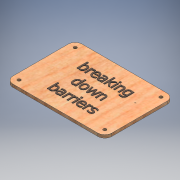
# Autodesk Inventor part: PromptPanel
Saved by Autodesk Inventor 2016 (Build 200138000, 138)
## iProperties
Created: 2015-09-18
Part Number: PromptPanel
Material: Generic
Document SubType Name: Modeling
Designer: Erin
Density: 1 g/cm^3
Appearance: Default
Author: Erin
Autodesk Inventor part; units mm, degrees
(part 1 of 2)
ref_plane "YZ Plane" through (0, 0, 0) normal (1, 0, 0) x (0, 1, 0)
ref_plane "XZ Plane" through (0, 0, 0) normal (0, 1, 0) x (-1, 0, 0)
ref_plane "XY Plane" through (0, 0, 0) normal (0, 0, 1) x (1, 0, 0)
derived "FrontPanel.ipt"
sketch "Sketch1" plane through (0, 0, 0) normal (0, 0, 1) x (1, 0, 0)
  line L0 (-60, 85) -> (60, 85)
  line L1 (60, 85) -> (60, -85)
  line L2 (60, -85) -> (-60, -85)
  line L3 (-60, -85) -> (-60, 85)
  line L4 (-50, 56.6301) -> (50, 56.6301)
  line L5 (50, 56.6301) -> (50, -13.3699)
  line L6 (50, -13.3699) -> (-50, -13.3699)
  line L7 (-50, -13.3699) -> (-50, 56.6301)
  circle A0 centre (-25, -55) radius 13.85
  circle A1 centre (-25, -24.425) radius 2.7
  circle A2 centre (25, -24.425) radius 2.7
  line L8 (-25, 85) -> (-25, -85) construction
  line L9 (-60, -55) -> (60, -55) construction
  circle A3 centre (-25, -55) radius 17.875 construction
  line L10 (25, 85) -> (25, -85) construction
  circle A4 centre (25, -55) radius 13.85
  circle A5 centre (25, -55) radius 17.875 construction
  circle A6 centre (-53.4, -78.4) radius 1.6
  line L11 (-52.9471, 75) -> (52.9471, 75) construction
  line L12 (52.9471, 75) -> (52.9471, 66.6301) construction
  line L13 (52.9471, 66.6301) -> (-52.9471, 66.6301) construction
  line L14 (-52.9471, 66.6301) -> (-52.9471, 75) construction
  circle A7 centre (-43.4, -6.7699) radius 1.6
  line L15 (-50, 21.6301) -> (50, 21.6301) construction
  line L16 (0, 56.6301) -> (0, -13.3699) construction
  circle A8 centre (-43.4, 50.0301) radius 1.6
  circle A9 centre (43.4, 50.0301) radius 1.6
  circle A10 centre (43.4, -6.7699) radius 1.6
  line L17 (-60, 0) -> (60, 0) construction
  circle A11 centre (53.4, -78.4) radius 1.6
  circle A12 centre (53.4, 78.4) radius 1.6
  circle A13 centre (-53.4, 78.4) radius 1.6
  point P0 (0, 0)
  point P1 (0, 85)
  point P2 (0, 75)
extrude "Extrusion1" add sketch "Sketch1" along normal blind 3 contours L4 L5 L6 L7
fillet "Fillet1" radius 7 4 edges at (-50, -13.3699, 1.5) (-50, 56.6301, 1.5) (50, 56.6301, 1.5) (50, -13.3699, 1.5)
sketch "Sketch2" plane through (-43, 56.6301, 3) normal (0, 0, 1) x (1, 0, 0)
  line L0 (25.4474, -13.3812) -> (62.0414, -13.3812) construction
  line L1 (62.0414, -13.3812) -> (62.0414, -43.8913) construction
  line L2 (62.0414, -43.8913) -> (25.4474, -43.8913) construction
  line L3 (25.4474, -43.8913) -> (25.4474, -13.3812) construction
  spline S0 degree 2 poles (24.8101, -19.9533) (24.8101, -21.7928) (23.0272, -24.0376) (21.682, -24.0376) knots 0 0 0 1 2 2 2
  spline S1 degree 2 poles (21.682, -24.0376) (21.0742, -24.0376) (20.2071, -23.7377) (19.7857, -23.4784) knots 0 0 0 1 2 2 2
  line L4 (19.7857, -23.4784) -> (19.7047, -23.8269)
  line L5 (19.7047, -23.8269) -> (18.5216, -23.8269)
  line L6 (18.5216, -23.8269) -> (18.5216, -13.3812)
  line L7 (18.5216, -13.3812) -> (19.7857, -13.3812)
  line L8 (19.7857, -13.3812) -> (19.7857, -17.1089)
  spline S2 degree 2 poles (19.7857, -17.1089) (20.2639, -16.6794) (21.3741, -16.1121) (22.0791, -16.1121) knots 0 0 0 1 2 2 2
  spline S3 degree 2 poles (22.0791, -16.1121) (23.3514, -16.1121) (24.8101, -18.1462) (24.8101, -19.9533) knots 0 0 0 1 2 2 2
  spline S4 degree 2 poles (23.5054, -20.0505) (23.5054, -18.7053) (22.6869, -17.3115) (21.7793, -17.3115) knots 0 0 0 1 2 2 2
  spline S5 degree 2 poles (21.7793, -17.3115) (21.2687, -17.3115) (20.2152, -17.7977) (19.7857, -18.1705) knots 0 0 0 1 2 2 2
  line L9 (19.7857, -18.1705) -> (19.7857, -22.4735)
  spline S6 degree 2 poles (19.7857, -22.4735) (20.2639, -22.7085) (21.0013, -22.903) (21.4389, -22.903) knots 0 0 0 1 2 2 2
  spline S7 degree 2 poles (21.4389, -22.903) (22.4032, -22.903) (23.5054, -21.5335) (23.5054, -20.0505) knots 0 0 0 1 2 2 2
  line L10 (30.1018, -17.6761) -> (30.037, -17.6761)
  spline S8 degree 2 poles (30.037, -17.6761) (29.8911, -17.6356) (29.575, -17.6194) (29.3562, -17.6194) knots 0 0 0 1 2 2 2
  spline S9 degree 2 poles (29.3562, -17.6194) (28.8457, -17.6194) (27.8408, -18.0651) (27.387, -18.5027) knots 0 0 0 1 2 2 2
  line L11 (27.387, -18.5027) -> (27.387, -23.8269)
  line L12 (27.387, -23.8269) -> (26.1229, -23.8269)
  line L13 (26.1229, -23.8269) -> (26.1229, -16.3228)
  line L14 (26.1229, -16.3228) -> (27.387, -16.3228)
  line L15 (27.387, -16.3228) -> (27.387, -17.4411)
  spline S10 degree 2 poles (27.387, -17.4411) (28.0759, -16.8252) (29.105, -16.3228) (29.5913, -16.3228) knots 0 0 0 1 2 2 2
  spline S11 degree 2 poles (29.5913, -16.3228) (29.7857, -16.3228) (29.9802, -16.339) (30.1018, -16.3633) knots 0 0 0 1 2 2 2
  line L16 (30.1018, -16.3633) -> (30.1018, -17.6761)
  spline S12 degree 2 poles (34.34, -23.997) (32.541, -23.997) (30.5637, -21.9792) (30.5637, -20.1154) knots 0 0 0 1 2 2 2
  spline S13 degree 2 poles (30.5637, -20.1154) (30.5637, -18.2839) (32.4843, -16.1121) (34.0321, -16.1121) knots 0 0 0 1 2 2 2
  spline S14 degree 2 poles (34.0321, -16.1121) (34.729, -16.1121) (35.8068, -16.5173) (36.2039, -16.9468) knots 0 0 0 1 2 2 2
  spline S15 degree 2 poles (36.2039, -16.9468) (36.6091, -17.3763) (37.0386, -18.6162) (37.0386, -19.5157) knots 0 0 0 1 2 2 2
  line L17 (37.0386, -19.5157) -> (37.0386, -20.2045)
  line L18 (37.0386, -20.2045) -> (31.8441, -20.2045)
  spline S16 degree 2 poles (31.8441, -20.2045) (31.8441, -21.5092) (33.1569, -22.8949) (34.3238, -22.8949) knots 0 0 0 1 2 2 2
  spline S17 degree 2 poles (34.3238, -22.8949) (34.7371, -22.8949) (35.5394, -22.7085) (35.8635, -22.5627) knots 0 0 0 1 2 2 2
  spline S18 degree 2 poles (35.8635, -22.5627) (36.2039, -22.4006) (36.6739, -22.117) (36.8279, -21.9873) knots 0 0 0 1 2 2 2
  line L19 (36.8279, -21.9873) -> (36.9008, -21.9873)
  line L20 (36.9008, -21.9873) -> (36.9008, -23.365)
  spline S19 degree 2 poles (36.9008, -23.365) (36.682, -23.4541) (36.0175, -23.7134) (35.7582, -23.7863) knots 0 0 0 1 2 2 2
  spline S20 degree 2 poles (35.7582, -23.7863) (35.3935, -23.8917) (34.7938, -23.997) (34.34, -23.997) knots 0 0 0 1 2 2 2
  spline S21 degree 2 poles (35.8068, -19.2402) (35.7906, -18.7296) (35.5799, -17.9841) (35.3773, -17.7329) knots 0 0 0 1 2 2 2
  spline S22 degree 2 poles (35.3773, -17.7329) (35.1585, -17.4492) (34.4697, -17.1494) (33.9592, -17.1494) knots 0 0 0 1 2 2 2
  spline S23 degree 2 poles (33.9592, -17.1494) (33.4567, -17.1494) (32.7517, -17.4492) (32.46, -17.741) knots 0 0 0 1 2 2 2
  spline S24 degree 2 poles (32.46, -17.741) (32.1763, -18.0408) (31.8846, -18.762) (31.8441, -19.2402) knots 0 0 0 1 2 2 2
  line L21 (31.8441, -19.2402) -> (35.8068, -19.2402)
  spline S25 degree 2 poles (42.5005, -23.0327) (42.3465, -23.1462) (41.8279, -23.5513) (41.5848, -23.6729) knots 0 0 0 1 2 2 2
  spline S26 degree 2 poles (41.5848, -23.6729) (41.2525, -23.8512) (40.6285, -24.0376) (40.0613, -24.0376) knots 0 0 0 1 2 2 2
  spline S27 degree 2 poles (40.0613, -24.0376) (39.5994, -24.0376) (38.7647, -23.6891) (38.4486, -23.3731) knots 0 0 0 1 2 2 2
  spline S28 degree 2 poles (38.4486, -23.3731) (38.1488, -23.0651) (37.7841, -22.1575) (37.7841, -21.6551) knots 0 0 0 1 2 2 2
  spline S29 degree 2 poles (37.7841, -21.6551) (37.7841, -20.8771) (38.4405, -19.775) (39.1537, -19.459) knots 0 0 0 1 2 2 2
  spline S30 degree 2 poles (39.1537, -19.459) (39.7857, -19.1672) (41.5037, -18.9484) (42.5005, -18.8917) knots 0 0 0 1 2 2 2
  line L22 (42.5005, -18.8917) -> (42.5005, -18.6486)
  spline S31 degree 2 poles (42.5005, -18.6486) (42.5005, -18.211) (42.2331, -17.668) (41.99, -17.5141) knots 0 0 0 1 2 2 2
  spline S32 degree 2 poles (41.99, -17.5141) (41.7468, -17.3601) (41.0499, -17.2628) (40.6772, -17.2628) knots 0 0 0 1 2 2 2
  spline S33 degree 2 poles (40.6772, -17.2628) (40.2396, -17.2628) (39.0564, -17.5222) (38.4648, -17.7734) knots 0 0 0 1 2 2 2
  line L23 (38.4648, -17.7734) -> (38.3919, -17.7734)
  line L24 (38.3919, -17.7734) -> (38.3919, -16.4849)
  spline S34 degree 2 poles (38.3919, -16.4849) (38.7404, -16.3876) (40.0451, -16.1445) (40.6853, -16.1445) knots 0 0 0 1 2 2 2
  spline S35 degree 2 poles (40.6853, -16.1445) (41.4632, -16.1445) (42.5248, -16.3876) (42.9462, -16.7037) knots 0 0 0 1 2 2 2
  spline S36 degree 2 poles (42.9462, -16.7037) (43.3595, -17.0116) (43.7647, -17.9922) (43.7647, -18.6972) knots 0 0 0 1 2 2 2
  line L25 (43.7647, -18.6972) -> (43.7647, -23.8269)
  line L26 (43.7647, -23.8269) -> (42.5005, -23.8269)
  line L27 (42.5005, -23.8269) -> (42.5005, -23.0327)
  line L28 (42.5005, -21.9792) -> (42.5005, -19.8966)
  spline S37 degree 2 poles (42.5005, -19.8966) (42.0467, -19.9371) (40.6772, -20.0748) (40.2477, -20.2045) knots 0 0 0 1 2 2 2
  spline S38 degree 2 poles (40.2477, -20.2045) (39.7452, -20.3585) (39.0888, -20.9987) (39.0888, -21.5659) knots 0 0 0 1 2 2 2
  spline S39 degree 2 poles (39.0888, -21.5659) (39.0888, -22.2142) (39.8182, -22.8706) (40.5151, -22.8706) knots 0 0 0 1 2 2 2
  spline S40 degree 2 poles (40.5151, -22.8706) (41.1066, -22.8706) (42.0791, -22.3601) (42.5005, -21.9792) knots 0 0 0 1 2 2 2
  line L29 (51.7549, -23.8269) -> (50.0937, -23.8269)
  line L30 (50.0937, -23.8269) -> (47.306, -20.2045)
  line L31 (47.306, -20.2045) -> (46.8036, -20.6907)
  line L32 (46.8036, -20.6907) -> (46.8036, -23.8269)
  line L33 (46.8036, -23.8269) -> (45.5394, -23.8269)
  line L34 (45.5394, -23.8269) -> (45.5394, -13.3812)
  line L35 (45.5394, -13.3812) -> (46.8036, -13.3812)
  line L36 (46.8036, -13.3812) -> (46.8036, -19.4914)
  line L37 (46.8036, -19.4914) -> (49.7695, -16.3228)
  line L38 (49.7695, -16.3228) -> (51.3417, -16.3228)
  line L39 (51.3417, -16.3228) -> (48.2622, -19.459)
  line L40 (48.2622, -19.459) -> (51.7549, -23.8269)
  line L41 (53.6755, -23.8269) -> (52.4113, -23.8269)
  line L42 (52.4113, -23.8269) -> (52.4113, -16.3228)
  line L43 (52.4113, -16.3228) -> (53.6755, -16.3228)
  line L44 (53.6755, -16.3228) -> (53.6755, -23.8269)
  line L45 (53.7647, -15.0748) -> (52.3303, -15.0748)
  line L46 (52.3303, -15.0748) -> (52.3303, -13.762)
  line L47 (52.3303, -13.762) -> (53.7647, -13.762)
  line L48 (53.7647, -13.762) -> (53.7647, -15.0748)
  line L49 (61.4227, -23.8269) -> (60.1585, -23.8269)
  line L50 (60.1585, -23.8269) -> (60.1585, -19.5481)
  spline S41 degree 2 poles (60.1585, -19.5481) (60.1585, -19.0295) (60.0613, -18.138) (59.9154, -17.8706) knots 0 0 0 1 2 2 2
  spline S42 degree 2 poles (59.9154, -17.8706) (59.7614, -17.587) (59.2104, -17.3115) (58.7404, -17.3115) knots 0 0 0 1 2 2 2
  spline S43 degree 2 poles (58.7404, -17.3115) (58.2703, -17.3115) (57.2736, -17.8139) (56.7955, -18.2191) knots 0 0 0 1 2 2 2
  line L51 (56.7955, -18.2191) -> (56.7955, -23.8269)
  line L52 (56.7955, -23.8269) -> (55.5313, -23.8269)
  line L53 (55.5313, -23.8269) -> (55.5313, -16.3228)
  line L54 (55.5313, -16.3228) -> (56.7955, -16.3228)
  line L55 (56.7955, -16.3228) -> (56.7955, -17.1575)
  spline S44 degree 2 poles (56.7955, -17.1575) (57.3627, -16.647) (58.4567, -16.1121) (59.0726, -16.1121) knots 0 0 0 1 2 2 2
  spline S45 degree 2 poles (59.0726, -16.1121) (60.1747, -16.1121) (61.4227, -17.5708) (61.4227, -18.9565) knots 0 0 0 1 2 2 2
  line L56 (61.4227, -18.9565) -> (61.4227, -23.8269)
  spline S46 degree 2 poles (63.4648, -25.0262) (63.5945, -25.0829) (64.0888, -25.2612) (64.4049, -25.3342) knots 0 0 0 1 2 2 2
  spline S47 degree 2 poles (64.4049, -25.3342) (64.7533, -25.4233) (65.3449, -25.5286) (65.6934, -25.5286) knots 0 0 0 1 2 2 2
  spline S48 degree 2 poles (65.6934, -25.5286) (66.2768, -25.5286) (67.0872, -25.2207) (67.3141, -24.9452) knots 0 0 0 1 2 2 2
  spline S49 degree 2 poles (67.3141, -24.9452) (67.5329, -24.6697) (67.7031, -23.9484) (67.7031, -23.4865) knots 0 0 0 1 2 2 2
  line L57 (67.7031, -23.4865) -> (67.7031, -22.8301)
  spline S50 degree 2 poles (67.7031, -22.8301) (67.1925, -23.2758) (66.212, -23.6972) (65.4746, -23.6972) knots 0 0 0 1 2 2 2
  spline S51 degree 2 poles (65.4746, -23.6972) (64.1942, -23.6972) (62.6788, -21.7928) (62.6788, -20.0019) knots 0 0 0 1 2 2 2
  spline S52 degree 2 poles (62.6788, -20.0019) (62.6788, -19.07) (63.2055, -17.6275) (63.6431, -17.117) knots 0 0 0 1 2 2 2
  spline S53 degree 2 poles (63.6431, -17.117) (64.0645, -16.6389) (65.2233, -16.1121) (65.8392, -16.1121) knots 0 0 0 1 2 2 2
  spline S54 degree 2 poles (65.8392, -16.1121) (66.4227, -16.1121) (67.2736, -16.3876) (67.7031, -16.6389) knots 0 0 0 1 2 2 2
  line L58 (67.7031, -16.6389) -> (67.776, -16.3228)
  line L59 (67.776, -16.3228) -> (68.9673, -16.3228)
  line L60 (68.9673, -16.3228) -> (68.9673, -22.9679)
  spline S55 degree 2 poles (68.9673, -22.9679) (68.9673, -24.8803) (67.306, -26.6632) (65.5961, -26.6632) knots 0 0 0 1 2 2 2
  spline S56 degree 2 poles (65.5961, -26.6632) (65.0451, -26.6632) (63.8943, -26.4849) (63.4, -26.339) knots 0 0 0 1 2 2 2
  line L61 (63.4, -26.339) -> (63.4, -25.0262)
  line L62 (63.4, -25.0262) -> (63.4648, -25.0262)
  line L63 (67.7031, -21.7928) -> (67.7031, -17.668)
  spline S57 degree 2 poles (67.7031, -17.668) (67.2331, -17.4411) (66.4389, -17.2466) (66.0418, -17.2466) knots 0 0 0 1 2 2 2
  spline S58 degree 2 poles (66.0418, -17.2466) (65.0856, -17.2466) (63.9835, -18.6567) (63.9835, -19.9776) knots 0 0 0 1 2 2 2
  spline S59 degree 2 poles (63.9835, -19.9776) (63.9835, -21.2256) (64.8182, -22.5303) (65.7582, -22.5303) knots 0 0 0 1 2 2 2
  spline S60 degree 2 poles (65.7582, -22.5303) (66.2525, -22.5303) (67.2898, -22.1413) (67.7031, -21.7928) knots 0 0 0 1 2 2 2
  line L64 (33.9632, -40.2916) -> (32.699, -40.2916)
  line L65 (32.699, -40.2916) -> (32.699, -39.5298)
  spline S61 degree 2 poles (32.699, -39.5298) (32.4073, -39.773) (31.9778, -40.0971) (31.6861, -40.2349) knots 0 0 0 1 2 2 2
  spline S62 degree 2 poles (31.6861, -40.2349) (31.4186, -40.3645) (30.8433, -40.5023) (30.4624, -40.5023) knots 0 0 0 1 2 2 2
  spline S63 degree 2 poles (30.4624, -40.5023) (29.8465, -40.5023) (28.8092, -39.9918) (28.4446, -39.4974) knots 0 0 0 1 2 2 2
  spline S64 degree 2 poles (28.4446, -39.4974) (28.0799, -39.0031) (27.6747, -37.5444) (27.6747, -36.5963) knots 0 0 0 1 2 2 2
  spline S65 degree 2 poles (27.6747, -36.5963) (27.6747, -35.6076) (28.1853, -34.1652) (28.631, -33.6222) knots 0 0 0 1 2 2 2
  spline S66 degree 2 poles (28.631, -33.6222) (29.0442, -33.136) (30.2031, -32.5769) (30.8433, -32.5769) knots 0 0 0 1 2 2 2
  spline S67 degree 2 poles (30.8433, -32.5769) (31.4024, -32.5769) (32.2371, -32.8281) (32.699, -33.0874) knots 0 0 0 1 2 2 2
  line L66 (32.699, -33.0874) -> (32.699, -29.8459)
  line L67 (32.699, -29.8459) -> (33.9632, -29.8459)
  line L68 (33.9632, -29.8459) -> (33.9632, -40.2916)
  line L69 (32.699, -38.4683) -> (32.699, -34.1328)
  spline S68 degree 2 poles (32.699, -34.1328) (32.229, -33.9059) (31.4835, -33.7357) (31.054, -33.7357) knots 0 0 0 1 2 2 2
  spline S69 degree 2 poles (31.054, -33.7357) (30.0815, -33.7357) (28.9794, -35.1944) (28.9794, -36.572) knots 0 0 0 1 2 2 2
  spline S70 degree 2 poles (28.9794, -36.572) (28.9794, -37.901) (29.8222, -39.3029) (30.7541, -39.3029) knots 0 0 0 1 2 2 2
  spline S71 degree 2 poles (30.7541, -39.3029) (31.2485, -39.3029) (32.2533, -38.8491) (32.699, -38.4683) knots 0 0 0 1 2 2 2
  spline S72 degree 2 poles (41.9616, -36.5396) (41.9616, -38.4358) (40.1383, -40.5023) (38.6148, -40.5023) knots 0 0 0 1 2 2 2
  spline S73 degree 2 poles (38.6148, -40.5023) (37.0507, -40.5023) (35.2598, -38.371) (35.2598, -36.5396) knots 0 0 0 1 2 2 2
  spline S74 degree 2 poles (35.2598, -36.5396) (35.2598, -34.6595) (37.1075, -32.5769) (38.6148, -32.5769) knots 0 0 0 1 2 2 2
  spline S75 degree 2 poles (38.6148, -32.5769) (40.1383, -32.5769) (41.9616, -34.6514) (41.9616, -36.5396) knots 0 0 0 1 2 2 2
  spline S76 degree 2 poles (40.6569, -36.5396) (40.6569, -35.0809) (39.5953, -33.6628) (38.6148, -33.6628) knots 0 0 0 1 2 2 2
  spline S77 degree 2 poles (38.6148, -33.6628) (37.6342, -33.6628) (36.5645, -35.0809) (36.5645, -36.5396) knots 0 0 0 1 2 2 2
  spline S78 degree 2 poles (36.5645, -36.5396) (36.5645, -37.9577) (37.6342, -39.4164) (38.6148, -39.4164) knots 0 0 0 1 2 2 2
  spline S79 degree 2 poles (38.6148, -39.4164) (39.5872, -39.4164) (40.6569, -37.982) (40.6569, -36.5396) knots 0 0 0 1 2 2 2
  line L70 (52.3506, -32.7875) -> (50.4462, -40.2916)
  line L71 (50.4462, -40.2916) -> (49.2793, -40.2916)
  line L72 (49.2793, -40.2916) -> (47.4478, -34.5055)
  line L73 (47.4478, -34.5055) -> (45.6245, -40.2916)
  line L74 (45.6245, -40.2916) -> (44.4656, -40.2916)
  line L75 (44.4656, -40.2916) -> (42.5451, -32.7875)
  line L76 (42.5451, -32.7875) -> (43.8579, -32.7875)
  line L77 (43.8579, -32.7875) -> (45.1869, -38.5979)
  line L78 (45.1869, -38.5979) -> (46.9616, -32.7875)
  line L79 (46.9616, -32.7875) -> (48.007, -32.7875)
  line L80 (48.007, -32.7875) -> (49.8303, -38.5979)
  line L81 (49.8303, -38.5979) -> (51.0783, -32.7875)
  line L82 (51.0783, -32.7875) -> (52.3506, -32.7875)
  line L83 (59.3522, -40.2916) -> (58.088, -40.2916)
  line L84 (58.088, -40.2916) -> (58.088, -36.0128)
  spline S80 degree 2 poles (58.088, -36.0128) (58.088, -35.4942) (57.9908, -34.6028) (57.8449, -34.3354) knots 0 0 0 1 2 2 2
  spline S81 degree 2 poles (57.8449, -34.3354) (57.6909, -34.0517) (57.1399, -33.7762) (56.6699, -33.7762) knots 0 0 0 1 2 2 2
  spline S82 degree 2 poles (56.6699, -33.7762) (56.1998, -33.7762) (55.2031, -34.2786) (54.725, -34.6838) knots 0 0 0 1 2 2 2
  line L85 (54.725, -34.6838) -> (54.725, -40.2916)
  line L86 (54.725, -40.2916) -> (53.4608, -40.2916)
  line L87 (53.4608, -40.2916) -> (53.4608, -32.7875)
  line L88 (53.4608, -32.7875) -> (54.725, -32.7875)
  line L89 (54.725, -32.7875) -> (54.725, -33.6222)
  spline S83 degree 2 poles (54.725, -33.6222) (55.2922, -33.1117) (56.3862, -32.5769) (57.0021, -32.5769) knots 0 0 0 1 2 2 2
  spline S84 degree 2 poles (57.0021, -32.5769) (58.1042, -32.5769) (59.3522, -34.0355) (59.3522, -35.4213) knots 0 0 0 1 2 2 2
  line L90 (59.3522, -35.4213) -> (59.3522, -40.2916)
  spline S85 degree 2 poles (27.8408, -52.8828) (27.8408, -54.7223) (26.058, -56.967) (24.7128, -56.967) knots 0 0 0 1 2 2 2
  spline S86 degree 2 poles (24.7128, -56.967) (24.105, -56.967) (23.2379, -56.6672) (22.8165, -56.4079) knots 0 0 0 1 2 2 2
  line L91 (22.8165, -56.4079) -> (22.7355, -56.7563)
  line L92 (22.7355, -56.7563) -> (21.5524, -56.7563)
  line L93 (21.5524, -56.7563) -> (21.5524, -46.3106)
  line L94 (21.5524, -46.3106) -> (22.8165, -46.3106)
  line L95 (22.8165, -46.3106) -> (22.8165, -50.0383)
  spline S87 degree 2 poles (22.8165, -50.0383) (23.2947, -49.6088) (24.4049, -49.0416) (25.1099, -49.0416) knots 0 0 0 1 2 2 2
  spline S88 degree 2 poles (25.1099, -49.0416) (26.3822, -49.0416) (27.8408, -51.0756) (27.8408, -52.8828) knots 0 0 0 1 2 2 2
  spline S89 degree 2 poles (26.5361, -52.98) (26.5361, -51.6348) (25.7177, -50.2409) (24.8101, -50.2409) knots 0 0 0 1 2 2 2
  spline S90 degree 2 poles (24.8101, -50.2409) (24.2995, -50.2409) (23.246, -50.7272) (22.8165, -51.0999) knots 0 0 0 1 2 2 2
  line L96 (22.8165, -51.0999) -> (22.8165, -55.403)
  spline S91 degree 2 poles (22.8165, -55.403) (23.2947, -55.638) (24.0321, -55.8325) (24.4697, -55.8325) knots 0 0 0 1 2 2 2
  spline S92 degree 2 poles (24.4697, -55.8325) (25.434, -55.8325) (26.5361, -54.463) (26.5361, -52.98) knots 0 0 0 1 2 2 2
  spline S93 degree 2 poles (33.3352, -55.9622) (33.1812, -56.0756) (32.6626, -56.4808) (32.4195, -56.6024) knots 0 0 0 1 2 2 2
  spline S94 degree 2 poles (32.4195, -56.6024) (32.0872, -56.7806) (31.4632, -56.967) (30.896, -56.967) knots 0 0 0 1 2 2 2
  spline S95 degree 2 poles (30.896, -56.967) (30.434, -56.967) (29.5994, -56.6186) (29.2833, -56.3025) knots 0 0 0 1 2 2 2
  spline S96 degree 2 poles (29.2833, -56.3025) (28.9835, -55.9946) (28.6188, -55.087) (28.6188, -54.5845) knots 0 0 0 1 2 2 2
  spline S97 degree 2 poles (28.6188, -54.5845) (28.6188, -53.8066) (29.2752, -52.7045) (29.9883, -52.3884) knots 0 0 0 1 2 2 2
  spline S98 degree 2 poles (29.9883, -52.3884) (30.6204, -52.0967) (32.3384, -51.8779) (33.3352, -51.8212) knots 0 0 0 1 2 2 2
  line L97 (33.3352, -51.8212) -> (33.3352, -51.5781)
  spline S99 degree 2 poles (33.3352, -51.5781) (33.3352, -51.1405) (33.0678, -50.5975) (32.8246, -50.4435) knots 0 0 0 1 2 2 2
  spline S100 degree 2 poles (32.8246, -50.4435) (32.5815, -50.2896) (31.8846, -50.1923) (31.5118, -50.1923) knots 0 0 0 1 2 2 2
  spline S101 degree 2 poles (31.5118, -50.1923) (31.0742, -50.1923) (29.8911, -50.4516) (29.2995, -50.7029) knots 0 0 0 1 2 2 2
  line L98 (29.2995, -50.7029) -> (29.2266, -50.7029)
  line L99 (29.2266, -50.7029) -> (29.2266, -49.4144)
  spline S102 degree 2 poles (29.2266, -49.4144) (29.575, -49.3171) (30.8797, -49.074) (31.5199, -49.074) knots 0 0 0 1 2 2 2
  spline S103 degree 2 poles (31.5199, -49.074) (32.2979, -49.074) (33.3595, -49.3171) (33.7809, -49.6332) knots 0 0 0 1 2 2 2
  spline S104 degree 2 poles (33.7809, -49.6332) (34.1942, -49.9411) (34.5994, -50.9217) (34.5994, -51.6267) knots 0 0 0 1 2 2 2
  line L100 (34.5994, -51.6267) -> (34.5994, -56.7563)
  line L101 (34.5994, -56.7563) -> (33.3352, -56.7563)
  line L102 (33.3352, -56.7563) -> (33.3352, -55.9622)
  line L103 (33.3352, -54.9087) -> (33.3352, -52.826)
  spline S105 degree 2 poles (33.3352, -52.826) (32.8814, -52.8665) (31.5118, -53.0043) (31.0823, -53.134) knots 0 0 0 1 2 2 2
  spline S106 degree 2 poles (31.0823, -53.134) (30.5799, -53.2879) (29.9235, -53.9281) (29.9235, -54.4954) knots 0 0 0 1 2 2 2
  spline S107 degree 2 poles (29.9235, -54.4954) (29.9235, -55.1437) (30.6528, -55.8001) (31.3498, -55.8001) knots 0 0 0 1 2 2 2
  spline S108 degree 2 poles (31.3498, -55.8001) (31.9413, -55.8001) (32.9138, -55.2896) (33.3352, -54.9087) knots 0 0 0 1 2 2 2
  line L104 (40.353, -50.6056) -> (40.2882, -50.6056)
  spline S109 degree 2 poles (40.2882, -50.6056) (40.1423, -50.5651) (39.8263, -50.5489) (39.6075, -50.5489) knots 0 0 0 1 2 2 2
  spline S110 degree 2 poles (39.6075, -50.5489) (39.0969, -50.5489) (38.0921, -50.9946) (37.6383, -51.4322) knots 0 0 0 1 2 2 2
  line L105 (37.6383, -51.4322) -> (37.6383, -56.7563)
  line L106 (37.6383, -56.7563) -> (36.3741, -56.7563)
  line L107 (36.3741, -56.7563) -> (36.3741, -49.2523)
  line L108 (36.3741, -49.2523) -> (37.6383, -49.2523)
  line L109 (37.6383, -49.2523) -> (37.6383, -50.3706)
  spline S111 degree 2 poles (37.6383, -50.3706) (38.3271, -49.7547) (39.3562, -49.2523) (39.8425, -49.2523) knots 0 0 0 1 2 2 2
  spline S112 degree 2 poles (39.8425, -49.2523) (40.037, -49.2523) (40.2314, -49.2685) (40.353, -49.2928) knots 0 0 0 1 2 2 2
  line L110 (40.353, -49.2928) -> (40.353, -50.6056)
  line L111 (45.3125, -50.6056) -> (45.2477, -50.6056)
  spline S113 degree 2 poles (45.2477, -50.6056) (45.1018, -50.5651) (44.7857, -50.5489) (44.5669, -50.5489) knots 0 0 0 1 2 2 2
  spline S114 degree 2 poles (44.5669, -50.5489) (44.0564, -50.5489) (43.0515, -50.9946) (42.5977, -51.4322) knots 0 0 0 1 2 2 2
  line L112 (42.5977, -51.4322) -> (42.5977, -56.7563)
  line L113 (42.5977, -56.7563) -> (41.3336, -56.7563)
  line L114 (41.3336, -56.7563) -> (41.3336, -49.2523)
  line L115 (41.3336, -49.2523) -> (42.5977, -49.2523)
  line L116 (42.5977, -49.2523) -> (42.5977, -50.3706)
  spline S115 degree 2 poles (42.5977, -50.3706) (43.2866, -49.7547) (44.3157, -49.2523) (44.8019, -49.2523) knots 0 0 0 1 2 2 2
  spline S116 degree 2 poles (44.8019, -49.2523) (44.9964, -49.2523) (45.1909, -49.2685) (45.3125, -49.2928) knots 0 0 0 1 2 2 2
  line L117 (45.3125, -49.2928) -> (45.3125, -50.6056)
  line L118 (47.5815, -56.7563) -> (46.3173, -56.7563)
  line L119 (46.3173, -56.7563) -> (46.3173, -49.2523)
  line L120 (46.3173, -49.2523) -> (47.5815, -49.2523)
  line L121 (47.5815, -49.2523) -> (47.5815, -56.7563)
  line L122 (47.6707, -48.0043) -> (46.2363, -48.0043)
  line L123 (46.2363, -48.0043) -> (46.2363, -46.6915)
  line L124 (46.2363, -46.6915) -> (47.6707, -46.6915)
  line L125 (47.6707, -46.6915) -> (47.6707, -48.0043)
  spline S117 degree 2 poles (52.695, -56.9265) (50.896, -56.9265) (48.9186, -54.9087) (48.9186, -53.0448) knots 0 0 0 1 2 2 2
  spline S118 degree 2 poles (48.9186, -53.0448) (48.9186, -51.2134) (50.8392, -49.0416) (52.387, -49.0416) knots 0 0 0 1 2 2 2
  spline S119 degree 2 poles (52.387, -49.0416) (53.084, -49.0416) (54.1618, -49.4468) (54.5588, -49.8763) knots 0 0 0 1 2 2 2
  spline S120 degree 2 poles (54.5588, -49.8763) (54.964, -50.3058) (55.3935, -51.5456) (55.3935, -52.4452) knots 0 0 0 1 2 2 2
  line L126 (55.3935, -52.4452) -> (55.3935, -53.134)
  line L127 (55.3935, -53.134) -> (50.199, -53.134)
  spline S121 degree 2 poles (50.199, -53.134) (50.199, -54.4387) (51.5118, -55.8244) (52.6788, -55.8244) knots 0 0 0 1 2 2 2
  spline S122 degree 2 poles (52.6788, -55.8244) (53.0921, -55.8244) (53.8943, -55.638) (54.2185, -55.4922) knots 0 0 0 1 2 2 2
  spline S123 degree 2 poles (54.2185, -55.4922) (54.5588, -55.3301) (55.0289, -55.0464) (55.1828, -54.9168) knots 0 0 0 1 2 2 2
  line L128 (55.1828, -54.9168) -> (55.2558, -54.9168)
  line L129 (55.2558, -54.9168) -> (55.2558, -56.2944)
  spline S124 degree 2 poles (55.2558, -56.2944) (55.037, -56.3836) (54.3725, -56.6429) (54.1131, -56.7158) knots 0 0 0 1 2 2 2
  spline S125 degree 2 poles (54.1131, -56.7158) (53.7485, -56.8212) (53.1488, -56.9265) (52.695, -56.9265) knots 0 0 0 1 2 2 2
  spline S126 degree 2 poles (54.1618, -52.1696) (54.1455, -51.6591) (53.9349, -50.9135) (53.7323, -50.6623) knots 0 0 0 1 2 2 2
  spline S127 degree 2 poles (53.7323, -50.6623) (53.5135, -50.3787) (52.8246, -50.0789) (52.3141, -50.0789) knots 0 0 0 1 2 2 2
  spline S128 degree 2 poles (52.3141, -50.0789) (51.8117, -50.0789) (51.1066, -50.3787) (50.8149, -50.6704) knots 0 0 0 1 2 2 2
  spline S129 degree 2 poles (50.8149, -50.6704) (50.5313, -50.9703) (50.2396, -51.6915) (50.199, -52.1696) knots 0 0 0 1 2 2 2
  line L130 (50.199, -52.1696) -> (54.1618, -52.1696)
  line L131 (60.6528, -50.6056) -> (60.588, -50.6056)
  spline S130 degree 2 poles (60.588, -50.6056) (60.4421, -50.5651) (60.1261, -50.5489) (59.9073, -50.5489) knots 0 0 0 1 2 2 2
  spline S131 degree 2 poles (59.9073, -50.5489) (59.3968, -50.5489) (58.3919, -50.9946) (57.9381, -51.4322) knots 0 0 0 1 2 2 2
  line L132 (57.9381, -51.4322) -> (57.9381, -56.7563)
  line L133 (57.9381, -56.7563) -> (56.6739, -56.7563)
  line L134 (56.6739, -56.7563) -> (56.6739, -49.2523)
  line L135 (56.6739, -49.2523) -> (57.9381, -49.2523)
  line L136 (57.9381, -49.2523) -> (57.9381, -50.3706)
  spline S132 degree 2 poles (57.9381, -50.3706) (58.6269, -49.7547) (59.6561, -49.2523) (60.1423, -49.2523) knots 0 0 0 1 2 2 2
  spline S133 degree 2 poles (60.1423, -49.2523) (60.3368, -49.2523) (60.5313, -49.2685) (60.6528, -49.2928) knots 0 0 0 1 2 2 2
  line L137 (60.6528, -49.2928) -> (60.6528, -50.6056)
  spline S134 degree 2 poles (63.6593, -56.9346) (62.9057, -56.9346) (61.601, -56.5294) (61.1715, -56.3025) knots 0 0 0 1 2 2 2
  line L138 (61.1715, -56.3025) -> (61.1715, -54.8844)
  line L139 (61.1715, -54.8844) -> (61.2363, -54.8844)
  spline S135 degree 2 poles (61.2363, -54.8844) (61.3984, -55.014) (61.836, -55.322) (62.2007, -55.4922) knots 0 0 0 1 2 2 2
  spline S136 degree 2 poles (62.2007, -55.4922) (62.5167, -55.6461) (63.2947, -55.873) (63.7079, -55.873) knots 0 0 0 1 2 2 2
  spline S137 degree 2 poles (63.7079, -55.873) (64.0078, -55.873) (64.6966, -55.7353) (64.8587, -55.6218) knots 0 0 0 1 2 2 2
  spline S138 degree 2 poles (64.8587, -55.6218) (65.0937, -55.4678) (65.3044, -55.1194) (65.3044, -54.7628) knots 0 0 0 1 2 2 2
  spline S139 degree 2 poles (65.3044, -54.7628) (65.3044, -54.3171) (64.8182, -53.8552) (64.1942, -53.7012) knots 0 0 0 1 2 2 2
  spline S140 degree 2 poles (64.1942, -53.7012) (63.9511, -53.6445) (63.1731, -53.4824) (62.8408, -53.3933) knots 0 0 0 1 2 2 2
  spline S141 degree 2 poles (62.8408, -53.3933) (61.9819, -53.1421) (61.2039, -52.1048) (61.2039, -51.3674) knots 0 0 0 1 2 2 2
  spline S142 degree 2 poles (61.2039, -51.3674) (61.2039, -50.3463) (62.7355, -49.074) (63.9997, -49.074) knots 0 0 0 1 2 2 2
  spline S143 degree 2 poles (63.9997, -49.074) (64.6237, -49.074) (65.8878, -49.3819) (66.3173, -49.617) knots 0 0 0 1 2 2 2
  line L140 (66.3173, -49.617) -> (66.3173, -50.9703)
  line L141 (66.3173, -50.9703) -> (66.2525, -50.9703)
  spline S144 degree 2 poles (66.2525, -50.9703) (65.7663, -50.5813) (64.5831, -50.1356) (63.9754, -50.1356) knots 0 0 0 1 2 2 2
  spline S145 degree 2 poles (63.9754, -50.1356) (63.3514, -50.1356) (62.4924, -50.6623) (62.4924, -51.1891) knots 0 0 0 1 2 2 2
  spline S146 degree 2 poles (62.4924, -51.1891) (62.4924, -51.6672) (63.0029, -52.1291) (63.5702, -52.275) knots 0 0 0 1 2 2 2
  spline S147 degree 2 poles (63.5702, -52.275) (63.8457, -52.3479) (64.5426, -52.4938) (64.9235, -52.5829) knots 0 0 0 1 2 2 2
  spline S148 degree 2 poles (64.9235, -52.5829) (65.7501, -52.7936) (66.5929, -53.758) (66.5929, -54.5926) knots 0 0 0 1 2 2 2
  spline S149 degree 2 poles (66.5929, -54.5926) (66.5929, -55.0789) (66.212, -55.9379) (65.8392, -56.2539) knots 0 0 0 1 2 2 2
  spline S150 degree 2 poles (65.8392, -56.2539) (65.4421, -56.5862) (64.4292, -56.9346) (63.6593, -56.9346) knots 0 0 0 1 2 2 2
  spline S151 degree 2 poles (24.8101, -19.9533) (24.8101, -21.7928) (23.0272, -24.0376) (21.682, -24.0376) knots 0 0 0 1 2 2 2
  spline S152 degree 2 poles (21.682, -24.0376) (21.0742, -24.0376) (20.2071, -23.7377) (19.7857, -23.4784) knots 0 0 0 1 2 2 2
  line L142 (19.7857, -23.4784) -> (19.7047, -23.8269)
  line L143 (19.7047, -23.8269) -> (18.5216, -23.8269)
  line L144 (18.5216, -23.8269) -> (18.5216, -13.3812)
  line L145 (18.5216, -13.3812) -> (19.7857, -13.3812)
  line L146 (19.7857, -13.3812) -> (19.7857, -17.1089)
  spline S153 degree 2 poles (19.7857, -17.1089) (20.2639, -16.6794) (21.3741, -16.1121) (22.0791, -16.1121) knots 0 0 0 1 2 2 2
  spline S154 degree 2 poles (22.0791, -16.1121) (23.3514, -16.1121) (24.8101, -18.1462) (24.8101, -19.9533) knots 0 0 0 1 2 2 2
  spline S155 degree 2 poles (23.5054, -20.0505) (23.5054, -18.7053) (22.6869, -17.3115) (21.7793, -17.3115) knots 0 0 0 1 2 2 2
  spline S156 degree 2 poles (21.7793, -17.3115) (21.2687, -17.3115) (20.2152, -17.7977) (19.7857, -18.1705) knots 0 0 0 1 2 2 2
  line L147 (19.7857, -18.1705) -> (19.7857, -22.4735)
  spline S157 degree 2 poles (19.7857, -22.4735) (20.2639, -22.7085) (21.0013, -22.903) (21.4389, -22.903) knots 0 0 0 1 2 2 2
  spline S158 degree 2 poles (21.4389, -22.903) (22.4032, -22.903) (23.5054, -21.5335) (23.5054, -20.0505) knots 0 0 0 1 2 2 2
  line L148 (30.1018, -17.6761) -> (30.037, -17.6761)
  spline S159 degree 2 poles (30.037, -17.6761) (29.8911, -17.6356) (29.575, -17.6194) (29.3562, -17.6194) knots 0 0 0 1 2 2 2
  spline S160 degree 2 poles (29.3562, -17.6194) (28.8457, -17.6194) (27.8408, -18.0651) (27.387, -18.5027) knots 0 0 0 1 2 2 2
  line L149 (27.387, -18.5027) -> (27.387, -23.8269)
  line L150 (27.387, -23.8269) -> (26.1229, -23.8269)
  line L151 (26.1229, -23.8269) -> (26.1229, -16.3228)
  line L152 (26.1229, -16.3228) -> (27.387, -16.3228)
  line L153 (27.387, -16.3228) -> (27.387, -17.4411)
  spline S161 degree 2 poles (27.387, -17.4411) (28.0759, -16.8252) (29.105, -16.3228) (29.5913, -16.3228) knots 0 0 0 1 2 2 2
  spline S162 degree 2 poles (29.5913, -16.3228) (29.7857, -16.3228) (29.9802, -16.339) (30.1018, -16.3633) knots 0 0 0 1 2 2 2
  line L154 (30.1018, -16.3633) -> (30.1018, -17.6761)
  spline S163 degree 2 poles (34.34, -23.997) (32.541, -23.997) (30.5637, -21.9792) (30.5637, -20.1154) knots 0 0 0 1 2 2 2
  spline S164 degree 2 poles (30.5637, -20.1154) (30.5637, -18.2839) (32.4843, -16.1121) (34.0321, -16.1121) knots 0 0 0 1 2 2 2
  spline S165 degree 2 poles (34.0321, -16.1121) (34.729, -16.1121) (35.8068, -16.5173) (36.2039, -16.9468) knots 0 0 0 1 2 2 2
  spline S166 degree 2 poles (36.2039, -16.9468) (36.6091, -17.3763) (37.0386, -18.6162) (37.0386, -19.5157) knots 0 0 0 1 2 2 2
  line L155 (37.0386, -19.5157) -> (37.0386, -20.2045)
  line L156 (37.0386, -20.2045) -> (31.8441, -20.2045)
  spline S167 degree 2 poles (31.8441, -20.2045) (31.8441, -21.5092) (33.1569, -22.8949) (34.3238, -22.8949) knots 0 0 0 1 2 2 2
  spline S168 degree 2 poles (34.3238, -22.8949) (34.7371, -22.8949) (35.5394, -22.7085) (35.8635, -22.5627) knots 0 0 0 1 2 2 2
  spline S169 degree 2 poles (35.8635, -22.5627) (36.2039, -22.4006) (36.6739, -22.117) (36.8279, -21.9873) knots 0 0 0 1 2 2 2
  line L157 (36.8279, -21.9873) -> (36.9008, -21.9873)
  line L158 (36.9008, -21.9873) -> (36.9008, -23.365)
  spline S170 degree 2 poles (36.9008, -23.365) (36.682, -23.4541) (36.0175, -23.7134) (35.7582, -23.7863) knots 0 0 0 1 2 2 2
  spline S171 degree 2 poles (35.7582, -23.7863) (35.3935, -23.8917) (34.7938, -23.997) (34.34, -23.997) knots 0 0 0 1 2 2 2
  spline S172 degree 2 poles (35.8068, -19.2402) (35.7906, -18.7296) (35.5799, -17.9841) (35.3773, -17.7329) knots 0 0 0 1 2 2 2
  spline S173 degree 2 poles (35.3773, -17.7329) (35.1585, -17.4492) (34.4697, -17.1494) (33.9592, -17.1494) knots 0 0 0 1 2 2 2
  spline S174 degree 2 poles (33.9592, -17.1494) (33.4567, -17.1494) (32.7517, -17.4492) (32.46, -17.741) knots 0 0 0 1 2 2 2
  spline S175 degree 2 poles (32.46, -17.741) (32.1763, -18.0408) (31.8846, -18.762) (31.8441, -19.2402) knots 0 0 0 1 2 2 2
  line L159 (31.8441, -19.2402) -> (35.8068, -19.2402)
  spline S176 degree 2 poles (42.5005, -23.0327) (42.3465, -23.1462) (41.8279, -23.5513) (41.5848, -23.6729) knots 0 0 0 1 2 2 2
  spline S177 degree 2 poles (41.5848, -23.6729) (41.2525, -23.8512) (40.6285, -24.0376) (40.0613, -24.0376) knots 0 0 0 1 2 2 2
  spline S178 degree 2 poles (40.0613, -24.0376) (39.5994, -24.0376) (38.7647, -23.6891) (38.4486, -23.3731) knots 0 0 0 1 2 2 2
  spline S179 degree 2 poles (38.4486, -23.3731) (38.1488, -23.0651) (37.7841, -22.1575) (37.7841, -21.6551) knots 0 0 0 1 2 2 2
  spline S180 degree 2 poles (37.7841, -21.6551) (37.7841, -20.8771) (38.4405, -19.775) (39.1537, -19.459) knots 0 0 0 1 2 2 2
  spline S181 degree 2 poles (39.1537, -19.459) (39.7857, -19.1672) (41.5037, -18.9484) (42.5005, -18.8917) knots 0 0 0 1 2 2 2
  line L160 (42.5005, -18.8917) -> (42.5005, -18.6486)
  spline S182 degree 2 poles (42.5005, -18.6486) (42.5005, -18.211) (42.2331, -17.668) (41.99, -17.5141) knots 0 0 0 1 2 2 2
  spline S183 degree 2 poles (41.99, -17.5141) (41.7468, -17.3601) (41.0499, -17.2628) (40.6772, -17.2628) knots 0 0 0 1 2 2 2
  spline S184 degree 2 poles (40.6772, -17.2628) (40.2396, -17.2628) (39.0564, -17.5222) (38.4648, -17.7734) knots 0 0 0 1 2 2 2
  line L161 (38.4648, -17.7734) -> (38.3919, -17.7734)
  line L162 (38.3919, -17.7734) -> (38.3919, -16.4849)
  spline S185 degree 2 poles (38.3919, -16.4849) (38.7404, -16.3876) (40.0451, -16.1445) (40.6853, -16.1445) knots 0 0 0 1 2 2 2
  spline S186 degree 2 poles (40.6853, -16.1445) (41.4632, -16.1445) (42.5248, -16.3876) (42.9462, -16.7037) knots 0 0 0 1 2 2 2
  spline S187 degree 2 poles (42.9462, -16.7037) (43.3595, -17.0116) (43.7647, -17.9922) (43.7647, -18.6972) knots 0 0 0 1 2 2 2
  line L163 (43.7647, -18.6972) -> (43.7647, -23.8269)
  line L164 (43.7647, -23.8269) -> (42.5005, -23.8269)
  line L165 (42.5005, -23.8269) -> (42.5005, -23.0327)
  line L166 (42.5005, -21.9792) -> (42.5005, -19.8966)
  spline S188 degree 2 poles (42.5005, -19.8966) (42.0467, -19.9371) (40.6772, -20.0748) (40.2477, -20.2045) knots 0 0 0 1 2 2 2
  spline S189 degree 2 poles (40.2477, -20.2045) (39.7452, -20.3585) (39.0888, -20.9987) (39.0888, -21.5659) knots 0 0 0 1 2 2 2
  spline S190 degree 2 poles (39.0888, -21.5659) (39.0888, -22.2142) (39.8182, -22.8706) (40.5151, -22.8706) knots 0 0 0 1 2 2 2
  spline S191 degree 2 poles (40.5151, -22.8706) (41.1066, -22.8706) (42.0791, -22.3601) (42.5005, -21.9792) knots 0 0 0 1 2 2 2
  line L167 (51.7549, -23.8269) -> (50.0937, -23.8269)
  line L168 (50.0937, -23.8269) -> (47.306, -20.2045)
  line L169 (47.306, -20.2045) -> (46.8036, -20.6907)
  line L170 (46.8036, -20.6907) -> (46.8036, -23.8269)
  line L171 (46.8036, -23.8269) -> (45.5394, -23.8269)
  line L172 (45.5394, -23.8269) -> (45.5394, -13.3812)
  line L173 (45.5394, -13.3812) -> (46.8036, -13.3812)
  line L174 (46.8036, -13.3812) -> (46.8036, -19.4914)
  line L175 (46.8036, -19.4914) -> (49.7695, -16.3228)
  line L176 (49.7695, -16.3228) -> (51.3417, -16.3228)
  line L177 (51.3417, -16.3228) -> (48.2622, -19.459)
  line L178 (48.2622, -19.459) -> (51.7549, -23.8269)
  line L179 (53.6755, -23.8269) -> (52.4113, -23.8269)
  line L180 (52.4113, -23.8269) -> (52.4113, -16.3228)
  line L181 (52.4113, -16.3228) -> (53.6755, -16.3228)
  line L182 (53.6755, -16.3228) -> (53.6755, -23.8269)
  line L183 (53.7647, -15.0748) -> (52.3303, -15.0748)
  line L184 (52.3303, -15.0748) -> (52.3303, -13.762)
  line L185 (52.3303, -13.762) -> (53.7647, -13.762)
  line L186 (53.7647, -13.762) -> (53.7647, -15.0748)
  line L187 (61.4227, -23.8269) -> (60.1585, -23.8269)
  line L188 (60.1585, -23.8269) -> (60.1585, -19.5481)
  spline S192 degree 2 poles (60.1585, -19.5481) (60.1585, -19.0295) (60.0613, -18.138) (59.9154, -17.8706) knots 0 0 0 1 2 2 2
  spline S193 degree 2 poles (59.9154, -17.8706) (59.7614, -17.587) (59.2104, -17.3115) (58.7404, -17.3115) knots 0 0 0 1 2 2 2
  spline S194 degree 2 poles (58.7404, -17.3115) (58.2703, -17.3115) (57.2736, -17.8139) (56.7955, -18.2191) knots 0 0 0 1 2 2 2
  line L189 (56.7955, -18.2191) -> (56.7955, -23.8269)
  line L190 (56.7955, -23.8269) -> (55.5313, -23.8269)
  line L191 (55.5313, -23.8269) -> (55.5313, -16.3228)
  line L192 (55.5313, -16.3228) -> (56.7955, -16.3228)
  line L193 (56.7955, -16.3228) -> (56.7955, -17.1575)
  spline S195 degree 2 poles (56.7955, -17.1575) (57.3627, -16.647) (58.4567, -16.1121) (59.0726, -16.1121) knots 0 0 0 1 2 2 2
  spline S196 degree 2 poles (59.0726, -16.1121) (60.1747, -16.1121) (61.4227, -17.5708) (61.4227, -18.9565) knots 0 0 0 1 2 2 2
  line L194 (61.4227, -18.9565) -> (61.4227, -23.8269)
  spline S197 degree 2 poles (63.4648, -25.0262) (63.5945, -25.0829) (64.0888, -25.2612) (64.4049, -25.3342) knots 0 0 0 1 2 2 2
  spline S198 degree 2 poles (64.4049, -25.3342) (64.7533, -25.4233) (65.3449, -25.5286) (65.6934, -25.5286) knots 0 0 0 1 2 2 2
  spline S199 degree 2 poles (65.6934, -25.5286) (66.2768, -25.5286) (67.0872, -25.2207) (67.3141, -24.9452) knots 0 0 0 1 2 2 2
  spline S200 degree 2 poles (67.3141, -24.9452) (67.5329, -24.6697) (67.7031, -23.9484) (67.7031, -23.4865) knots 0 0 0 1 2 2 2
  line L195 (67.7031, -23.4865) -> (67.7031, -22.8301)
  spline S201 degree 2 poles (67.7031, -22.8301) (67.1925, -23.2758) (66.212, -23.6972) (65.4746, -23.6972) knots 0 0 0 1 2 2 2
  spline S202 degree 2 poles (65.4746, -23.6972) (64.1942, -23.6972) (62.6788, -21.7928) (62.6788, -20.0019) knots 0 0 0 1 2 2 2
  spline S203 degree 2 poles (62.6788, -20.0019) (62.6788, -19.07) (63.2055, -17.6275) (63.6431, -17.117) knots 0 0 0 1 2 2 2
  spline S204 degree 2 poles (63.6431, -17.117) (64.0645, -16.6389) (65.2233, -16.1121) (65.8392, -16.1121) knots 0 0 0 1 2 2 2
  spline S205 degree 2 poles (65.8392, -16.1121) (66.4227, -16.1121) (67.2736, -16.3876) (67.7031, -16.6389) knots 0 0 0 1 2 2 2
  line L196 (67.7031, -16.6389) -> (67.776, -16.3228)
  line L197 (67.776, -16.3228) -> (68.9673, -16.3228)
  line L198 (68.9673, -16.3228) -> (68.9673, -22.9679)
  spline S206 degree 2 poles (68.9673, -22.9679) (68.9673, -24.8803) (67.306, -26.6632) (65.5961, -26.6632) knots 0 0 0 1 2 2 2
  spline S207 degree 2 poles (65.5961, -26.6632) (65.0451, -26.6632) (63.8943, -26.4849) (63.4, -26.339) knots 0 0 0 1 2 2 2
  line L199 (63.4, -26.339) -> (63.4, -25.0262)
  line L200 (63.4, -25.0262) -> (63.4648, -25.0262)
  line L201 (67.7031, -21.7928) -> (67.7031, -17.668)
  spline S208 degree 2 poles (67.7031, -17.668) (67.2331, -17.4411) (66.4389, -17.2466) (66.0418, -17.2466) knots 0 0 0 1 2 2 2
  spline S209 degree 2 poles (66.0418, -17.2466) (65.0856, -17.2466) (63.9835, -18.6567) (63.9835, -19.9776) knots 0 0 0 1 2 2 2
  spline S210 degree 2 poles (63.9835, -19.9776) (63.9835, -21.2256) (64.8182, -22.5303) (65.7582, -22.5303) knots 0 0 0 1 2 2 2
  spline S211 degree 2 poles (65.7582, -22.5303) (66.2525, -22.5303) (67.2898, -22.1413) (67.7031, -21.7928) knots 0 0 0 1 2 2 2
  line L202 (33.9632, -40.2916) -> (32.699, -40.2916)
  line L203 (32.699, -40.2916) -> (32.699, -39.5298)
  spline S212 degree 2 poles (32.699, -39.5298) (32.4073, -39.773) (31.9778, -40.0971) (31.6861, -40.2349) knots 0 0 0 1 2 2 2
  spline S213 degree 2 poles (31.6861, -40.2349) (31.4186, -40.3645) (30.8433, -40.5023) (30.4624, -40.5023) knots 0 0 0 1 2 2 2
  spline S214 degree 2 poles (30.4624, -40.5023) (29.8465, -40.5023) (28.8092, -39.9918) (28.4446, -39.4974) knots 0 0 0 1 2 2 2
  spline S215 degree 2 poles (28.4446, -39.4974) (28.0799, -39.0031) (27.6747, -37.5444) (27.6747, -36.5963) knots 0 0 0 1 2 2 2
  spline S216 degree 2 poles (27.6747, -36.5963) (27.6747, -35.6076) (28.1853, -34.1652) (28.631, -33.6222) knots 0 0 0 1 2 2 2
  spline S217 degree 2 poles (28.631, -33.6222) (29.0442, -33.136) (30.2031, -32.5769) (30.8433, -32.5769) knots 0 0 0 1 2 2 2
  spline S218 degree 2 poles (30.8433, -32.5769) (31.4024, -32.5769) (32.2371, -32.8281) (32.699, -33.0874) knots 0 0 0 1 2 2 2
  line L204 (32.699, -33.0874) -> (32.699, -29.8459)
  line L205 (32.699, -29.8459) -> (33.9632, -29.8459)
  line L206 (33.9632, -29.8459) -> (33.9632, -40.2916)
  line L207 (32.699, -38.4683) -> (32.699, -34.1328)
  spline S219 degree 2 poles (32.699, -34.1328) (32.229, -33.9059) (31.4835, -33.7357) (31.054, -33.7357) knots 0 0 0 1 2 2 2
  spline S220 degree 2 poles (31.054, -33.7357) (30.0815, -33.7357) (28.9794, -35.1944) (28.9794, -36.572) knots 0 0 0 1 2 2 2
  spline S221 degree 2 poles (28.9794, -36.572) (28.9794, -37.901) (29.8222, -39.3029) (30.7541, -39.3029) knots 0 0 0 1 2 2 2
  spline S222 degree 2 poles (30.7541, -39.3029) (31.2485, -39.3029) (32.2533, -38.8491) (32.699, -38.4683) knots 0 0 0 1 2 2 2
  spline S223 degree 2 poles (41.9616, -36.5396) (41.9616, -38.4358) (40.1383, -40.5023) (38.6148, -40.5023) knots 0 0 0 1 2 2 2
  spline S224 degree 2 poles (38.6148, -40.5023) (37.0507, -40.5023) (35.2598, -38.371) (35.2598, -36.5396) knots 0 0 0 1 2 2 2
  spline S225 degree 2 poles (35.2598, -36.5396) (35.2598, -34.6595) (37.1075, -32.5769) (38.6148, -32.5769) knots 0 0 0 1 2 2 2
  spline S226 degree 2 poles (38.6148, -32.5769) (40.1383, -32.5769) (41.9616, -34.6514) (41.9616, -36.5396) knots 0 0 0 1 2 2 2
  spline S227 degree 2 poles (40.6569, -36.5396) (40.6569, -35.0809) (39.5953, -33.6628) (38.6148, -33.6628) knots 0 0 0 1 2 2 2
  spline S228 degree 2 poles (38.6148, -33.6628) (37.6342, -33.6628) (36.5645, -35.0809) (36.5645, -36.5396) knots 0 0 0 1 2 2 2
  spline S229 degree 2 poles (36.5645, -36.5396) (36.5645, -37.9577) (37.6342, -39.4164) (38.6148, -39.4164) knots 0 0 0 1 2 2 2
  spline S230 degree 2 poles (38.6148, -39.4164) (39.5872, -39.4164) (40.6569, -37.982) (40.6569, -36.5396) knots 0 0 0 1 2 2 2
  line L208 (52.3506, -32.7875) -> (50.4462, -40.2916)
  line L209 (50.4462, -40.2916) -> (49.2793, -40.2916)
  line L210 (49.2793, -40.2916) -> (47.4478, -34.5055)
  line L211 (47.4478, -34.5055) -> (45.6245, -40.2916)
  line L212 (45.6245, -40.2916) -> (44.4656, -40.2916)
  line L213 (44.4656, -40.2916) -> (42.5451, -32.7875)
  line L214 (42.5451, -32.7875) -> (43.8579, -32.7875)
  line L215 (43.8579, -32.7875) -> (45.1869, -38.5979)
  line L216 (45.1869, -38.5979) -> (46.9616, -32.7875)
  line L217 (46.9616, -32.7875) -> (48.007, -32.7875)
  line L218 (48.007, -32.7875) -> (49.8303, -38.5979)
  line L219 (49.8303, -38.5979) -> (51.0783, -32.7875)
  line L220 (51.0783, -32.7875) -> (52.3506, -32.7875)
  line L221 (59.3522, -40.2916) -> (58.088, -40.2916)
  line L222 (58.088, -40.2916) -> (58.088, -36.0128)
  spline S231 degree 2 poles (58.088, -36.0128) (58.088, -35.4942) (57.9908, -34.6028) (57.8449, -34.3354) knots 0 0 0 1 2 2 2
  spline S232 degree 2 poles (57.8449, -34.3354) (57.6909, -34.0517) (57.1399, -33.7762) (56.6699, -33.7762) knots 0 0 0 1 2 2 2
  spline S233 degree 2 poles (56.6699, -33.7762) (56.1998, -33.7762) (55.2031, -34.2786) (54.725, -34.6838) knots 0 0 0 1 2 2 2
  line L223 (54.725, -34.6838) -> (54.725, -40.2916)
  line L224 (54.725, -40.2916) -> (53.4608, -40.2916)
  line L225 (53.4608, -40.2916) -> (53.4608, -32.7875)
  line L226 (53.4608, -32.7875) -> (54.725, -32.7875)
  line L227 (54.725, -32.7875) -> (54.725, -33.6222)
  spline S234 degree 2 poles (54.725, -33.6222) (55.2922, -33.1117) (56.3862, -32.5769) (57.0021, -32.5769) knots 0 0 0 1 2 2 2
  spline S235 degree 2 poles (57.0021, -32.5769) (58.1042, -32.5769) (59.3522, -34.0355) (59.3522, -35.4213) knots 0 0 0 1 2 2 2
  line L228 (59.3522, -35.4213) -> (59.3522, -40.2916)
  spline S236 degree 2 poles (27.8408, -52.8828) (27.8408, -54.7223) (26.058, -56.967) (24.7128, -56.967) knots 0 0 0 1 2 2 2
  spline S237 degree 2 poles (24.7128, -56.967) (24.105, -56.967) (23.2379, -56.6672) (22.8165, -56.4079) knots 0 0 0 1 2 2 2
  line L229 (22.8165, -56.4079) -> (22.7355, -56.7563)
  line L230 (22.7355, -56.7563) -> (21.5524, -56.7563)
  line L231 (21.5524, -56.7563) -> (21.5524, -46.3106)
  line L232 (21.5524, -46.3106) -> (22.8165, -46.3106)
  line L233 (22.8165, -46.3106) -> (22.8165, -50.0383)
  spline S238 degree 2 poles (22.8165, -50.0383) (23.2947, -49.6088) (24.4049, -49.0416) (25.1099, -49.0416) knots 0 0 0 1 2 2 2
  spline S239 degree 2 poles (25.1099, -49.0416) (26.3822, -49.0416) (27.8408, -51.0756) (27.8408, -52.8828) knots 0 0 0 1 2 2 2
  spline S240 degree 2 poles (26.5361, -52.98) (26.5361, -51.6348) (25.7177, -50.2409) (24.8101, -50.2409) knots 0 0 0 1 2 2 2
  spline S241 degree 2 poles (24.8101, -50.2409) (24.2995, -50.2409) (23.246, -50.7272) (22.8165, -51.0999) knots 0 0 0 1 2 2 2
  line L234 (22.8165, -51.0999) -> (22.8165, -55.403)
  spline S242 degree 2 poles (22.8165, -55.403) (23.2947, -55.638) (24.0321, -55.8325) (24.4697, -55.8325) knots 0 0 0 1 2 2 2
  spline S243 degree 2 poles (24.4697, -55.8325) (25.434, -55.8325) (26.5361, -54.463) (26.5361, -52.98) knots 0 0 0 1 2 2 2
  spline S244 degree 2 poles (33.3352, -55.9622) (33.1812, -56.0756) (32.6626, -56.4808) (32.4195, -56.6024) knots 0 0 0 1 2 2 2
  spline S245 degree 2 poles (32.4195, -56.6024) (32.0872, -56.7806) (31.4632, -56.967) (30.896, -56.967) knots 0 0 0 1 2 2 2
  spline S246 degree 2 poles (30.896, -56.967) (30.434, -56.967) (29.5994, -56.6186) (29.2833, -56.3025) knots 0 0 0 1 2 2 2
  spline S247 degree 2 poles (29.2833, -56.3025) (28.9835, -55.9946) (28.6188, -55.087) (28.6188, -54.5845) knots 0 0 0 1 2 2 2
  spline S248 degree 2 poles (28.6188, -54.5845) (28.6188, -53.8066) (29.2752, -52.7045) (29.9883, -52.3884) knots 0 0 0 1 2 2 2
  spline S249 degree 2 poles (29.9883, -52.3884) (30.6204, -52.0967) (32.3384, -51.8779) (33.3352, -51.8212) knots 0 0 0 1 2 2 2
  line L235 (33.3352, -51.8212) -> (33.3352, -51.5781)
  spline S250 degree 2 poles (33.3352, -51.5781) (33.3352, -51.1405) (33.0678, -50.5975) (32.8246, -50.4435) knots 0 0 0 1 2 2 2
  spline S251 degree 2 poles (32.8246, -50.4435) (32.5815, -50.2896) (31.8846, -50.1923) (31.5118, -50.1923) knots 0 0 0 1 2 2 2
  spline S252 degree 2 poles (31.5118, -50.1923) (31.0742, -50.1923) (29.8911, -50.4516) (29.2995, -50.7029) knots 0 0 0 1 2 2 2
  line L236 (29.2995, -50.7029) -> (29.2266, -50.7029)
  line L237 (29.2266, -50.7029) -> (29.2266, -49.4144)
  spline S253 degree 2 poles (29.2266, -49.4144) (29.575, -49.3171) (30.8797, -49.074) (31.5199, -49.074) knots 0 0 0 1 2 2 2
  spline S254 degree 2 poles (31.5199, -49.074) (32.2979, -49.074) (33.3595, -49.3171) (33.7809, -49.6332) knots 0 0 0 1 2 2 2
  spline S255 degree 2 poles (33.7809, -49.6332) (34.1942, -49.9411) (34.5994, -50.9217) (34.5994, -51.6267) knots 0 0 0 1 2 2 2
  line L238 (34.5994, -51.6267) -> (34.5994, -56.7563)
  line L239 (34.5994, -56.7563) -> (33.3352, -56.7563)
  line L240 (33.3352, -56.7563) -> (33.3352, -55.9622)
  line L241 (33.3352, -54.9087) -> (33.3352, -52.826)
  spline S256 degree 2 poles (33.3352, -52.826) (32.8814, -52.8665) (31.5118, -53.0043) (31.0823, -53.134) knots 0 0 0 1 2 2 2
  spline S257 degree 2 poles (31.0823, -53.134) (30.5799, -53.2879) (29.9235, -53.9281) (29.9235, -54.4954) knots 0 0 0 1 2 2 2
  spline S258 degree 2 poles (29.9235, -54.4954) (29.9235, -55.1437) (30.6528, -55.8001) (31.3498, -55.8001) knots 0 0 0 1 2 2 2
  spline S259 degree 2 poles (31.3498, -55.8001) (31.9413, -55.8001) (32.9138, -55.2896) (33.3352, -54.9087) knots 0 0 0 1 2 2 2
  line L242 (40.353, -50.6056) -> (40.2882, -50.6056)
  spline S260 degree 2 poles (40.2882, -50.6056) (40.1423, -50.5651) (39.8263, -50.5489) (39.6075, -50.5489) knots 0 0 0 1 2 2 2
  spline S261 degree 2 poles (39.6075, -50.5489) (39.0969, -50.5489) (38.0921, -50.9946) (37.6383, -51.4322) knots 0 0 0 1 2 2 2
  line L243 (37.6383, -51.4322) -> (37.6383, -56.7563)
  line L244 (37.6383, -56.7563) -> (36.3741, -56.7563)
  line L245 (36.3741, -56.7563) -> (36.3741, -49.2523)
  line L246 (36.3741, -49.2523) -> (37.6383, -49.2523)
  line L247 (37.6383, -49.2523) -> (37.6383, -50.3706)
  spline S262 degree 2 poles (37.6383, -50.3706) (38.3271, -49.7547) (39.3562, -49.2523) (39.8425, -49.2523) knots 0 0 0 1 2 2 2
  spline S263 degree 2 poles (39.8425, -49.2523) (40.037, -49.2523) (40.2314, -49.2685) (40.353, -49.2928) knots 0 0 0 1 2 2 2
  line L248 (40.353, -49.2928) -> (40.353, -50.6056)
  line L249 (45.3125, -50.6056) -> (45.2477, -50.6056)
  spline S264 degree 2 poles (45.2477, -50.6056) (45.1018, -50.5651) (44.7857, -50.5489) (44.5669, -50.5489) knots 0 0 0 1 2 2 2